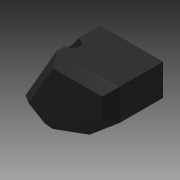
# Autodesk Inventor part: TSOP Holder Corner
Saved by Autodesk Inventor 2015 (Build 190159000, 159)
## iProperties
Created: 2015-11-27
Part Number: TSOP Holder Corner
Material: ABS Plastic
Document SubType Name: Modeling
Designer: James
Density: 1.06 g/cm^3
Appearance: Smooth - White
Author: James
Autodesk Inventor part; units mm, degrees
ref_plane "YZ Plane" through (0, 0, 0) normal (1, 0, 0) x (0, 1, 0)
ref_plane "XZ Plane" through (0, 0, 0) normal (0, 1, 0) x (-1, 0, 0)
ref_plane "XY Plane" through (0, 0, 0) normal (0, 0, 1) x (1, 0, 0)
sketch "Sketch1" plane through (0, 0, 0) normal (0, 1, 0) x (-1, 0, 0)
  line L0 (50.7332, 97.4522) -> (55.4964, 94.7022)
  line L1 (55.4964, 94.7022) -> (57.5964, 98.3395)
  line L2 (48.0701, 103.8395) -> (45.9701, 100.2022)
  line L3 (45.9701, 100.2022) -> (50.7332, 97.4522)
  arc A0 (55.0378, 99.8167) -> (50.6287, 102.3623) centre (52.3832, 100.3101) ccw
  line L4 (48.0701, 103.8395) -> (50.6287, 102.3623)
  line L5 (55.0378, 99.8167) -> (57.5964, 98.3395)
  line L6 (47.7332, 92.256) -> (54.0309, 89.9639)
  line L7 (47.7332, 92.256) -> (54.435, 92.256) construction
  line L8 (56.5464, 96.5209) -> (59.5464, 96.5209) construction
  line L9 (58.0464, 93.9228) -> (60.2464, 93.9228) construction
  line L10 (54.0309, 89.9639) -> (54.9868, 89.616)
  line L11 (55.2332, 105.2464) -> (61.9398, 93.6303)
  circle A1 centre (58.3542, 93.0522) radius 1.4
  line L12 (61.9398, 93.6303) -> (62.4398, 92.7643)
  line L13 (62.4398, 92.7643) -> (56.2134, 89.1695)
  line L14 (54.9868, 89.616) -> (56.2134, 89.1695)
  line L15 (47.7332, 92.256) -> (42.5993, 96.5639)
  line L16 (47.7332, 92.256) -> (44.3823, 98.06) construction
  line L17 (47.0201, 102.0209) -> (45.5201, 104.6189) construction
  line L18 (44.0201, 102.0209) -> (42.9201, 103.9261) construction
  line L19 (42.5993, 96.5639) -> (41.8201, 97.2178)
  line L20 (55.2332, 105.2464) -> (41.8201, 105.2464)
  circle A2 centre (43.1122, 101.8522) radius 1.4
  line L21 (41.8201, 105.2464) -> (40.8201, 105.2464)
  line L22 (40.8201, 105.2464) -> (40.8201, 98.0569)
  line L23 (41.8201, 97.2178) -> (40.8201, 98.0569)
  dimension "d8" = 20
  dimension "d26" = 2.8
  dimension "d27" = 1
  dimension "d31" = 2.8
  constraints: 48 end point, 3 centre point, 3 horizontal, 2 point on circle, 1 equal length, 1 midpoint, 1 perpendicular
  measures "d8" angle of L6 L7
  measures "d26" diameter of A1
  measures "d27" distance of L11.end L12.end
  measures "d31" diameter of A2
extrude "Extrusion1" add sketch "Sketch1" along normal blind 12
sketch "Sketch3" plane through (0, 0, 0) normal (0, -1, 0) x (1, 0, 0)
  line L0 (-48.0701, 103.8395) -> (-45.9701, 100.2022) projected
  line L1 (-45.9701, 100.2022) -> (-55.4964, 94.7022) projected
  line L2 (-55.4964, 94.7022) -> (-57.5964, 98.3395) projected
  line L3 (-57.5964, 98.3395) -> (-55.0378, 99.8167) projected
  arc A0 (-50.6287, 102.3623) -> (-55.0378, 99.8167) centre (-52.3832, 100.3101) ccw projected
  line L4 (-50.6287, 102.3623) -> (-48.0701, 103.8395) projected
  line L5 (-55.2332, 105.2464) -> (-62.4398, 92.7643) projected
  line L6 (-56.2134, 89.1695) -> (-47.7332, 92.256) projected
  line L7 (-62.4398, 92.7643) -> (-56.2134, 89.1695) projected
  line L8 (-47.7332, 92.256) -> (-40.8201, 98.0569) projected
  line L9 (-40.8201, 98.0569) -> (-40.8201, 105.2464) projected
  line L10 (-40.8201, 105.2464) -> (-55.2332, 105.2464) projected
  circle A1 centre (-58.3542, 93.0522) radius 1.4 projected
  circle A2 centre (-43.1122, 101.8522) radius 1.4 projected
  point P0 (0, 0)
extrude "Extrusion2" add sketch "Sketch3" against normal blind 2 contours L0 L1 L2 L3 A0 L4 | A1 | A2
sketch "Sketch4" plane through (-45.9701, 2, 100.2022) normal (-0.5, 0, 0.8660254) x (0.8660254, 0, 0.5)
  line L0 (0, 0) -> (-5.5, 0)
  line L1 (-11, 0) -> (0, 0) projected
  line L2 (-5.5, 0) -> (-5.5, 3.3)
  circle A0 centre (-5.5, 3.3) radius 1.5
  point P0 (-10.2898, -2)
  dimension "d21" = 3.3
  dimension "d22" = 3
  constraints: 4 end point, 1 centre point, 1 coincident, 1 midpoint, 1 perpendicular
  measures "d21" distance of L0.end L2.end
  measures "d22" diameter of A0
extrude "Extrusion3" cut sketch "Sketch4" along normal through all
chamfer "Chamfer2" distance 2 angle 45 6 edges at (-58.8365, 0, 99.0054) (-48.0267, 0, 105.2464) (-40.8201, 0, 101.6516) (-44.2767, 0, 95.1565) (-51.9733, 0, 90.7128) (-59.3266, 0, 90.9669)
body "Solid1"
